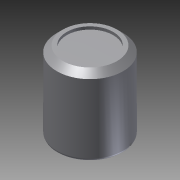
# Autodesk Inventor part: SB4011NOM-body
Saved by Autodesk Inventor 2014 (Build 180170000, 170)
## iProperties
Category: PARTsolutions
Company: NKKSWITCHES
Created: 2013-12-28
Part Number: SB4011NOM-body
Catalog Web Link: www.cadenas.de
Description: SB4011 Series - 3 Amp Momentary Pushbuttons -body-
Vendor: NKKSWITCHES
Document SubType Name: Modeling
Designer: PARTuser1
Manufacturer: NKKSWITCHES
Density: 1 g/cm^3
Material: Generic
Appearance: RGB(192.00000375509219,192.00000375509219,192.00000375509219)
PSOL_IDENT_0: {$CADENAS_DATA\23d-libs\nkkswitches\pushbuttons\sb4011\parts\sb4011_body.prj},227 {VTYP=3D},{NB=SB40
PSOL_IDENT_1: 11NOM-body},{LINA=SB4011NOM-body},{NN=SB4011 Series - 3 Amp Momentary Pushbuttons -body},{DATE=24.05
PSOL_IDENT_2: .2013 11:21:52},{GEOMDATE=24.05.2013 13:21:00},{VERSION=},{LINEID=10},{LINESUBID=-1},{WBVAR=PLSCRCTS
PSOL_IDENT_3: ,BSHNG}  {NB=SB4011NOM-body},{LINA=SB4011NOM-body},{KT=DUMMY},{PN=SB4011NOM},{SRS=SB40},{PLSCRCTS=11
PSOL_IDENT_4: NO},{BSHNG=M},{L=0.35400},{ND=0.47244},{C=0.19800}
CNS_NN: SB4011 Series - 3 Amp Momentary Pushbuttons -body
CNS_NB: SB4011NOM-body
CNS_NBSYN: $PN.-body
CNS_LINA: SB4011NOM-body
CNS_PN: SB4011NOM
CNS_SRS: SB40
CNS_PLSCRCTS: 11NO - SPST/OFF/(ON) (Normally Open)
CNS_BSHNG: M - Metric Threaded M12 P1
CNS_L: 0.35400
CNS_ND: 0.47244
CNS_C: 0.19800
SUPPLIER: NKKSWITCHES
ARTICLENO: SB4011NOM-body
BOMINFO: SB4011NOM-body
CREATOR: CADENAS GmbH
Title: SB4011NOM-body
Author: Cadenas PARTsolutions
Autodesk Inventor part; units mm, degrees
sketch "Sketch_2" plane through (0, 0, 0) normal (1, 0, 0) x (0, 1, 0)
  line L0 (0, 0) -> (8.9916, 0)
  line L1 (8.4836, 0) -> (8.4836, -4.2037)
  line L2 (8.4836, -4.2037) -> (8.9916, -4.2037)
  line L3 (8.9916, -4.2037) -> (8.9916, -4.9265)
  line L4 (8.9916, -4.9265) -> (7.9181, -6)
  line L5 (7.9181, -6) -> (0, -6)
  line L6 (0, -6) -> (0, 0)
  line L7 (0, 0) -> (8.4836, 0)
  constraints: 16 end point
revolve "Revolution1" add sketch "Sketch_2" angle 360 about axis through (0, 0, 0) along (0, -1, 0)
sketch "Sketch_3" plane through (0, 0, 0) normal (1, 0, 0) x (0, 1, 0)
  line L0 (-5.0292, 0) -> (0, 0)
  line L1 (0, 0) -> (0, -6)
  line L2 (0, -6) -> (-4.5212, -6)
  arc A0 (-5.0292, -5.492) -> (-4.5212, -6) centre (-4.5212, -5.492) ccw
  line L3 (-5.0292, -5.492) -> (-5.0292, 0)
  line L4 (-5.0292, 0) -> (0, 0)
  constraints: 10 end point, 2 point on circle, 1 centre point
revolve "Revolution2" add sketch "Sketch_3" angle 360 about axis through (0, -5.0292, 0) along (0, -1, 0)
sketch "Sketch_7" plane through (0, 0, 0) normal (1, 0, 0) x (0, 1, 0)
  line L0 (-5.2832, 0) -> (-0.254, 0)
  line L1 (-0.254, 0) -> (-0.254, -5.7404)
  line L2 (-0.254, -5.7404) -> (-4.2672, -5.7404)
  arc A0 (-4.7752, -5.2324) -> (-4.2672, -5.7404) centre (-4.2672, -5.2324) ccw
  line L3 (-4.7752, -5.2324) -> (-4.7752, -4.9784)
  line L4 (-4.7752, -4.9784) -> (-5.2832, -4.9784)
  line L5 (-5.2832, -4.9784) -> (-5.2832, 0)
  line L6 (-5.2832, 0) -> (-0.254, 0)
  constraints: 14 end point, 2 point on circle, 1 centre point
sketch "Sketch_9" plane through (0, -5.0292, 0) normal (0, 1, 0) x (1, 0, 0)
  line L0 (-11.646, -2.8576) -> (-11.5146, -3.3483)
  line L1 (-11.5146, -3.3483) -> (11.646, 2.8576)
  line L2 (11.646, 2.8576) -> (11.5146, 3.3483)
  line L3 (11.5146, 3.3483) -> (-11.646, -2.8576)
  constraints: 8 end point
extrude "Extrusion1" cut sketch "Sketch_9" along normal blind 0.762
revolve "Revolution3" cut sketch "Sketch_7" angle 360 about axis through (0, -5.2832, 0) along (0, -1, 0)
ref_plane "to_at504_knurled_face_nut_XY" through (0, 2.5146, 0) normal (0, -1, 0) x (1, 0, 0)
ref_plane "to_at504_knurled_face_nut_YZ" through (0, 2.5146, 0) normal (1, 0, 0) x (0, 0, 1)
ref_plane "to_at504_knurled_face_nut_ZX" through (0, 2.5146, 0) normal (0, 0, 1) x (0, -1, 0)
ref_plane "to_at508_lockwasher_XY" through (0, 2.0066, 0) normal (0, 1, 0) x (1, 0, 0)
ref_plane "to_at508_lockwasher_YZ" through (0, 2.0066, 0) normal (1, 0, 0) x (0, 0, -1)
ref_plane "to_at508_lockwasher_ZX" through (0, 2.0066, 0) normal (0, 0, -1) x (0, 1, 0)
ref_plane "to_dummy_XY" through (0, 0, 0) normal (0, -1, 0) x (1, 0, 0)
ref_plane "to_dummy_YZ" through (0, 0, 0) normal (1, 0, 0) x (0, 0, 1)
ref_plane "to_dummy_ZX" through (0, 0, 0) normal (0, 0, 1) x (0, -1, 0)
ref_plane "to_hex_nut_XY" through (0, 0, 0) normal (0, 1, 0) x (1, 0, 0)
ref_plane "to_hex_nut_YZ" through (0, 0, 0) normal (1, 0, 0) x (0, 0, -1)
ref_plane "to_hex_nut_ZX" through (0, 0, 0) normal (0, 0, -1) x (0, 1, 0)
ref_plane "to_plunger_XY" through (0, 8.9916, 0) normal (0, -1, 0) x (1, 0, 0)
ref_plane "to_plunger_YZ" through (0, 8.9916, 0) normal (1, 0, 0) x (0, 0, 1)
ref_plane "to_plunger_ZX" through (0, 8.9916, 0) normal (0, 0, 1) x (0, -1, 0)
ref_plane "to_trmnl_hold_XY" through (0, -5.0292, 0) normal (0, 1, 0) x (1, 0, 0)
ref_plane "to_trmnl_hold_YZ" through (0, -5.0292, 0) normal (1, 0, 0) x (0, 0, -1)
ref_plane "to_trmnl_hold_ZX" through (0, -5.0292, 0) normal (0, 0, -1) x (0, 1, 0)
body "Solid1"
